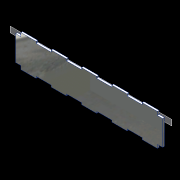
# Autodesk Inventor part: BottomPlateMiddle
Saved by Autodesk Inventor 2022 (Build 260153000, 153)
## iProperties
Created: 2022-04-18
Part Number: BottomPlateMiddle
Material: Aluminum 6061
Document SubType Name: Modeling
Designer: tandu
Density: 2.7 g/cm^3
Appearance: Aluminum - Flat
Author: tandu
Autodesk Inventor part; units mm, degrees
ref_plane "YZ Plane" through (0, 0, 0) normal (1, 0, 0) x (0, 1, 0)
ref_plane "XZ Plane" through (0, 0, 0) normal (0, 1, 0) x (-1, 0, 0)
ref_plane "XY Plane" through (0, 0, 0) normal (0, 0, 1) x (1, 0, 0)
ref_plane "Work Plane1" through (0, 0, 0) normal (0, 0, 1) x (1, 0, 0)
sketch "Sketch1" plane through (0, 0, 0) normal (0, 0, 1) x (1, 0, 0)
  line L0 (-1003.3, 38.1008) -> (-893.9926, 38.1008) construction
  line L1 (-893.9926, 38.1008) -> (-893.9926, 50.8008) projected
  line L2 (-1003.3, 50.8008) -> (-893.9926, 50.8008) projected
  line L3 (-1003.3, 38.1008) -> (-1003.3, 50.8008) projected
  line L4 (-893.9926, 38.1008) -> (-784.6248, 38.1008) projected
  line L5 (-784.6248, 38.1008) -> (-784.6248, 50.8008) projected
  line L6 (-893.9926, 50.8008) -> (-784.6248, 50.8008) projected
  line L7 (-893.9926, 38.1008) -> (-893.9926, 50.8008) projected
  line L8 (-784.6248, 38.1008) -> (-675.2569, 38.1008) construction
  line L9 (-675.2569, 38.1008) -> (-675.2569, 50.8008) projected
  line L10 (-784.6248, 50.8008) -> (-675.2569, 50.8008) projected
  line L11 (-784.6248, 38.1008) -> (-784.6248, 50.8008) projected
  line L12 (-675.2569, 38.1008) -> (-565.8891, 38.1008) projected
  line L13 (-565.8891, 38.1008) -> (-565.8891, 50.8008) projected
  line L14 (-675.2569, 50.8008) -> (-565.8891, 50.8008) projected
  line L15 (-675.2569, 38.1008) -> (-675.2569, 50.8008) projected
  line L16 (-565.8891, 38.1008) -> (-456.5213, 38.1008) construction
  line L17 (-456.5213, 38.1008) -> (-456.5213, 50.8008) projected
  line L18 (-565.8891, 50.8008) -> (-456.5213, 50.8008) projected
  line L19 (-565.8891, 38.1008) -> (-565.8891, 50.8008) projected
  line L20 (-456.5213, 38.1008) -> (-347.1535, 38.1008) projected
  line L21 (-347.1535, 38.1008) -> (-347.1535, 50.8008) projected
  line L22 (-456.5213, 50.8008) -> (-347.1535, 50.8008) projected
  line L23 (-456.5213, 38.1008) -> (-456.5213, 50.8008) projected
  line L24 (-347.1535, 38.1008) -> (-237.7856, 38.1008) construction
  line L25 (-237.7856, 38.1008) -> (-237.7856, 50.8008) projected
  line L26 (-347.1535, 50.8008) -> (-237.7856, 50.8008) projected
  line L27 (-347.1535, 38.1008) -> (-347.1535, 50.8008) projected
  line L28 (-237.7856, 38.1008) -> (-128.4178, 38.1008) projected
  line L29 (-128.4178, 38.1008) -> (-128.4178, 50.8008) projected
  line L30 (-237.7856, 50.8008) -> (-128.4178, 50.8008) projected
  line L31 (-237.7856, 38.1008) -> (-237.7856, 50.8008) projected
  line L32 (-128.4178, 38.1008) -> (-19.05, 38.1008) construction
  line L33 (-19.05, 38.1008) -> (-19.05, 50.8008) projected
  line L34 (-128.4178, 50.8008) -> (-19.05, 50.8008) projected
  line L35 (-128.4178, 38.1008) -> (-128.4178, 50.8008) projected
  line L36 (-128.4178, -180.9742) -> (-19.05, -180.9742) projected
  line L37 (-19.05, -180.9742) -> (-19.05, -168.2742) projected
  line L38 (-128.4178, -168.2742) -> (-19.05, -168.2742) construction
  line L39 (-128.4178, -180.9742) -> (-128.4178, -168.2742) projected
  line L40 (-237.7856, -180.9742) -> (-128.4178, -180.9742) projected
  line L41 (-128.4178, -180.9742) -> (-128.4178, -168.2742) projected
  line L42 (-237.7856, -168.2742) -> (-128.4178, -168.2742) projected
  line L43 (-237.7856, -180.9742) -> (-237.7856, -168.2742) projected
  line L44 (-347.1535, -180.9742) -> (-237.7856, -180.9742) projected
  line L45 (-237.7856, -180.9742) -> (-237.7856, -168.2742) projected
  line L46 (-347.1535, -168.2742) -> (-237.7856, -168.2742) construction
  line L47 (-347.1535, -180.9742) -> (-347.1535, -168.2742) projected
  line L48 (-456.5213, -180.9742) -> (-347.1535, -180.9742) projected
  line L49 (-347.1535, -180.9742) -> (-347.1535, -168.2742) projected
  line L50 (-456.5213, -168.2742) -> (-347.1535, -168.2742) projected
  line L51 (-456.5213, -180.9742) -> (-456.5213, -168.2742) projected
  line L52 (-675.2569, -180.9742) -> (-565.8891, -180.9742) projected
  line L53 (-565.8891, -180.9742) -> (-565.8891, -168.2742) projected
  line L54 (-675.2569, -168.2742) -> (-565.8891, -168.2742) projected
  line L55 (-675.2569, -180.9742) -> (-675.2569, -168.2742) projected
  line L56 (-893.9926, -180.9742) -> (-784.6248, -180.9742) projected
  line L57 (-784.6248, -180.9742) -> (-784.6248, -168.2742) projected
  line L58 (-893.9926, -168.2742) -> (-784.6248, -168.2742) projected
  line L59 (-893.9926, -180.9742) -> (-893.9926, -168.2742) projected
  line L60 (-1003.3, -180.9742) -> (-893.9926, -180.9742) projected
  line L61 (-893.9926, -180.9742) -> (-893.9926, -168.2742) projected
  line L62 (-1003.3, -168.2742) -> (-893.9926, -168.2742) construction
  line L63 (-1003.3, -180.9742) -> (-1003.3, -168.2742) projected
  line L64 (-784.6248, -180.9742) -> (-675.2569, -180.9742) projected
  line L65 (-675.2569, -180.9742) -> (-675.2569, -168.2742) projected
  line L66 (-784.6248, -168.2742) -> (-675.2569, -168.2742) construction
  line L67 (-784.6248, -180.9742) -> (-784.6248, -168.2742) projected
  line L68 (-565.8891, -180.9742) -> (-456.5213, -180.9742) projected
  line L69 (-456.5213, -180.9742) -> (-456.5213, -168.2742) projected
  line L70 (-565.8891, -168.2742) -> (-456.5213, -168.2742) construction
  line L71 (-565.8891, -180.9742) -> (-565.8891, -168.2742) projected
  line L72 (-1003.3, 38.1008) -> (-1003.3, -168.2742) construction
  line L73 (-19.05, 38.1008) -> (-19.05, -168.2742) construction
  line L74 (19.05, -130.175) -> (19.05, -241.3) projected
  line L75 (-19.05, -180.9742) -> (19.05, -180.9742)
  line L76 (19.05, -180.9742) -> (19.05, 50.8008)
  line L77 (19.05, 50.8008) -> (-19.05, 50.8008)
  line L78 (-19.05, 50.8008) -> (-19.05, -180.9742) construction
  line L79 (-1041.4, 0) -> (-1041.4, 285.75) projected
  line L80 (-1003.3, 50.8008) -> (-1041.4, 50.8008)
  line L81 (-1003.3, -180.9742) -> (-1041.4, -180.9742)
  line L82 (-1041.4, -180.9742) -> (-1041.4, 50.8008)
  line L83 (19.05, 0) -> (-1041.4, 0) construction
  line L84 (-1041.4, -130.175) -> (19.05, -130.175) construction
  line L85 (-1041.4, 50.8008) -> (-1003.3, 50.8008)
  line L86 (-1003.3, 50.8008) -> (-1003.3, 0)
  line L87 (-1003.3, 0) -> (-1041.4, 0) construction
  line L88 (-1041.4, 0) -> (-1041.4, 50.8008)
  line L89 (-1041.4, -180.9742) -> (-1003.3, -180.9742)
  line L90 (-1003.3, -180.9742) -> (-1003.3, -130.175)
  line L91 (-1003.3, -130.175) -> (-1041.4, -130.175) construction
  line L92 (-1041.4, -130.175) -> (-1041.4, -180.9742)
  line L93 (19.05, -180.9742) -> (-19.05, -180.9742)
  line L94 (-19.05, -180.9742) -> (-19.05, -130.175)
  line L95 (-19.05, -130.175) -> (19.05, -130.175) construction
  line L96 (19.05, -130.175) -> (19.05, -180.9742)
  line L97 (19.05, 50.8008) -> (-19.05, 50.8008)
  line L98 (-19.05, 50.8008) -> (-19.05, 0)
  line L99 (-19.05, 0) -> (19.05, 0) construction
  line L100 (19.05, 0) -> (19.05, 50.8008)
  line L101 (-1041.4, 25.4004) -> (-1003.3, 25.4004)
  line L102 (-1041.4, -155.5746) -> (-1003.3, -155.5746)
  line L103 (-1003.3, -180.9742) -> (-1003.3, -155.5746)
  line L104 (-19.05, -155.5746) -> (19.05, -155.5746)
  line L105 (-19.05, 25.4004) -> (19.05, 25.4004)
  point P0 (0, 0)
  constraints: 60 end point, 11 parallel, 10 point on line, 8 midpoint, 6 horizontal, 6 perpendicular, 3 collinear, 1 vertical
extrude "Base" add sketch "Sketch1" along normal blind 12.7 contours L4 L5 L10 L9 L12 L13 L18 L17 L20 L21 L26 L25 L28 L29 L34 L33 L98 L105 L76 L74 L104 L94 L37 L36 L39 L42 L43 L44 L47 L50 L51 L68 L53 L54 L55 L64 L57 L58 L59 L60 L63 L90 L102 L82 L79 L101 L86 L3 L2 L1
sketch "Sketch2" plane through (0, 0, 0) normal (0, 0, -1) x (-1, 0, 0)
  line L0 (-19.05, -155.5746) -> (-19.05, 25.4004) projected
  circle A0 centre (69.85, -39.6515) radius 3.2664
  circle A1 centre (69.85, -90.4515) radius 3.2664
  circle A2 centre (0, -39.6515) radius 3.2664
  circle A3 centre (0, -90.4515) radius 3.2664
  line L1 (76.2, -99.2501) -> (76.2, -30.9241)
  line L2 (76.2, -30.9241) -> (-19.05, -30.9241)
  line L3 (-19.05, -99.2501) -> (-19.05, -30.9241)
  line L4 (76.2, -99.2501) -> (-19.05, -99.2501)
  line L5 (-19.05, -155.5746) -> (-19.05, 25.4004) construction
  circle A4 centre (952.5, -90.5227) radius 3.2664
  circle A5 centre (952.5, -39.7227) radius 3.2664
  circle A6 centre (1022.35, -90.5227) radius 3.2664
  circle A7 centre (1022.35, -39.7227) radius 3.2664
  line L6 (946.15, -30.9241) -> (946.15, -99.2501)
  line L7 (946.15, -99.2501) -> (1041.4, -99.2501)
  line L8 (1041.4, -30.9241) -> (1041.4, -99.2501)
  line L9 (946.15, -30.9241) -> (1041.4, -30.9241)
  line L10 (1041.4, 25.4004) -> (1041.4, -155.5746) projected
  circle A8 centre (95.9501, -376.5553) radius 3.2664
  circle A9 centre (95.9501, -325.7553) radius 3.2664
  circle A10 centre (165.8001, -376.5553) radius 3.2664
  circle A11 centre (165.8001, -325.7553) radius 3.2664
  line L11 (89.6001, -316.9568) -> (89.6001, -385.2828)
  line L12 (89.6001, -385.2828) -> (184.8501, -385.2828)
  line L13 (184.8501, -316.9568) -> (184.8501, -385.2828)
  line L14 (89.6001, -316.9568) -> (184.8501, -316.9568)
  point P0 (0, 0)
  point P1 (-19.05, -65.0871)
  point P2 (1041.4, -65.0871)
  dimension "d13" = 68.326
  dimension "d14" = 95.25
  dimension "d15" = 6.5329
  dimension "d16" = 6.35
  dimension "d17" = 8.7986
  dimension "d18" = 8.7274
  dimension "d19" = 6.35
  dimension "d20" = 8.7274
  dimension "d21" = 19.05
  dimension "d22" = 19.05
  dimension "d23" = 8.7986
  dimension "d37" = 68.326
  dimension "d38" = 95.25
  dimension "d39" = 6.5329
  dimension "d40" = 6.35
  dimension "d41" = 8.7986
  dimension "d42" = 8.7274
  dimension "d43" = 6.35
  dimension "d44" = 8.7274
  dimension "d45" = 19.05
  dimension "d46" = 19.05
  dimension "d47" = 8.7986
  dimension "d48" = 68.326
  dimension "d49" = 95.25
  dimension "d50" = 6.5329
  dimension "d51" = 6.35
  dimension "d52" = 8.7986
  dimension "d53" = 8.7274
  dimension "d54" = 6.35
  dimension "d55" = 8.7274
  dimension "d56" = 19.05
  dimension "d57" = 19.05
  dimension "d58" = 8.7986
  constraints: 24 end point, 12 centre point, 9 equal radius, 6 perpendicular, 4 midpoint, 3 parallel, 2 collinear
  measures "d13" distance of L1.start L1.end
  measures "d14" distance of L1.start L3.start
  measures "d15" diameter of A1
  measures "d16" distance from line of L1 A1.centre
  measures "d17" distance from line of L4 A1.centre
  measures "d18" distance from line of L2 A0.centre
  measures "d19" distance from line of L1 A0.centre
  measures "d20" distance from line of L2 A2.centre
  measures "d21" distance from line of L3 A2.centre
  measures "d22" distance from line of L3 A3.centre
  measures "d23" distance from line of L4 A3.centre
  measures "d37" distance of L6.start L6.end
  measures "d38" distance of L6.start L8.start
  measures "d39" diameter of A5
  measures "d40" distance from line of L6 A5.centre
  measures "d41" distance from line of L9 A5.centre
  measures "d42" distance from line of L7 A4.centre
  measures "d43" distance from line of L6 A4.centre
  measures "d44" distance from line of L7 A6.centre
  measures "d45" distance from line of L8 A6.centre
  measures "d46" distance from line of L8 A7.centre
  measures "d47" distance from line of L9 A7.centre
  measures "d48" distance of L14.start L11.end
  measures "d49" distance of L14.start L13.start
  measures "d50" diameter of A9
  measures "d51" distance from line of L11 A9.centre
  measures "d52" distance from line of L14 A9.centre
  measures "d53" distance from line of L12 A8.centre
  measures "d54" distance from line of L11 A8.centre
  measures "d55" distance from line of L12 A10.centre
  measures "d56" distance from line of L13 A10.centre
  measures "d57" distance from line of L13 A11.centre
  measures "d58" distance from line of L14 A11.centre
extrude "DriveMotorHoles" cut sketch "Sketch2" against normal through all contours A0 | A1 | A2 | A3 | A4 | A5 | A6 | A7
equation "\"d0\" = Thickness"
equation "\"Thickness\" = 12.7"
body "Solid1"
